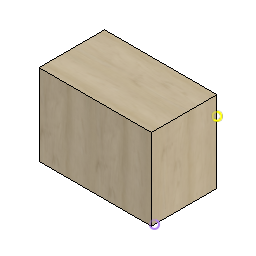
Laminar Casing. v4 (Autodesk Fusion 360 design; units mm, degrees)
Autodesk Fusion 360 part; units mm, degrees
sketch "Sketch1" plane through (0, 0, 0) normal (0, 0, 1) x (1, 0, 0)
  line L0 (25.4, 25.4) -> (939.8, 25.4)
  line L1 (939.8, 25.4) -> (939.8, 533.4)
  line L2 (939.8, 533.4) -> (25.4, 533.4)
  line L3 (25.4, 533.4) -> (25.4, 25.4)
  line L4 (101.6, 381) -> (863.6, 381)
  line L5 (863.6, 381) -> (863.6, 25.4)
  line L6 (863.6, 25.4) -> (101.6, 25.4)
  line L7 (101.6, 25.4) -> (101.6, 381)
  constraint horizontal L0
  constraint vertical L1
  constraint horizontal L2
  constraint vertical L3
  constraint horizontal L4
  constraint vertical L5
  constraint horizontal L6
  constraint vertical L7
  constraint coincident L0 L5.end
extrude "Extrude1" add sketch "Sketch1" against normal blind 508 contours L0 L1 L2 L3 L4 L5 L7
sketch "Sketch2" plane through (0, 0, 0) normal (0, 0, 1) x (1, 0, 0)
  point P0 (939.8, 25.4)
sketch "Sketch3" plane through (0, 0, 0) normal (0, 1, 0) x (1, 0, 0)
  line L0 (939.8, 508) -> (25.4, 508)
  line L1 (25.4, 508) -> (25.4, 0)
  line L2 (25.4, 0) -> (939.8, 0)
  line L3 (939.8, 0) -> (939.8, 508)
  constraint horizontal L0
  constraint vertical L1
  constraint horizontal L2
  constraint vertical L3
extrude "Extrude2" add sketch "Sketch3" along normal blind 25.4
sketch "Sketch4" plane through (0, 0, 0) normal (0, 0, 1) x (1, 0, 0)
box "BoxPrimitive1" add length 533.4 width 914.4 height 152.4 placed x (0, -1, 0) y (1, 0, 0) z (0, 0, 1) at (25.4, 533.4, 0)
sketch "Sketch5" plane through (0, 0, 0) normal (0, 1, 0) x (1, 0, 0)
sketch "Sketch6" plane through (0, 0, 0) normal (0, 0, 1) x (1, 0, 0)
  point P0 (939.8, 533.4)
fillet "Fillet1" radius 24.5618 3 edges at (482.6, 381, -508) (863.6, 203.2, -508) (101.6, 203.2, -508) 1 faces at (609.6, 262.4667, 0)
extrude "Extrude3" add 1 faces at (617.7873, 490.7873, -508) along direction (0, 0, 1) blind 12.7
ref_plane "WorkPlane2" through (482.6, 266.7, -177.8) normal (-1, 0, 0) x (0, 1, 0)
sketch "Sketch7" plane through (0, 533.4, 0) normal (0, 1, 0) x (-1, 0, 0)
  line L0 (-25.4, -508) -> (-25.4, 152.4)
  line L1 (-25.4, 152.4) -> (-939.8, 152.4)
  line L2 (-939.8, 152.4) -> (-939.8, -508)
  line L3 (-939.8, -508) -> (-25.4, -508)
  circle A0 centre (-482.6, -139.7) radius 114.3
  dimension "d14" = 228.6
  measures "d14" diameter of A0
extrude "Extrude4" cut sketch "Sketch7" against normal blind 12.7 contours A0
sketch "Sketch8" plane through (0, 0, 0) normal (0, 0, -1) x (1, 0, 0)
  line L0 (126.1618, -49.9618) -> (126.1618, -356.4382)
  line L1 (126.1618, -356.4382) -> (839.0382, -356.4382)
  line L2 (839.0382, -356.4382) -> (839.0382, -49.9618)
  line L3 (839.0382, -49.9618) -> (126.1618, -49.9618)
  line L4 (622.3, -114.3) -> (342.9, -114.3)
  arc A0 (342.9, -114.3) -> (342.9, -139.7) centre (342.9, -127) ccw
  line L5 (342.9, -139.7) -> (622.3, -139.7)
  arc A1 (622.3, -139.7) -> (622.3, -114.3) centre (622.3, -127) ccw
  line L6 (622.3, -127) -> (342.9, -127) construction
  point P0 (482.6, -127)
  constraint tangent L4 A0
  constraint tangent A0 L5
  constraint parallel L4 L5
  constraint tangent L5 A1
  constraint tangent L4 A1
  constraint parallel L1 L6
  constraint midpoint L6 P0
extrude "Extrude5" cut sketch "Sketch8" against normal blind 12.7 contours L4 A0 L5 A1
sketch "Sketch9" plane through (0, 381, 0) normal (0, -1, 0) x (1, 0, 0)
  line L0 (863.6, -24.5618) -> (101.6, -24.5618)
  line L1 (101.6, -24.5618) -> (101.6, -483.4382)
  line L2 (101.6, -483.4382) -> (863.6, -483.4382)
  line L3 (863.6, -483.4382) -> (863.6, -24.5618)
  line L4 (812.8, -50.8) -> (558.8, -50.8)
  arc A0 (558.8, -50.8) -> (558.8, -101.6) centre (558.8, -76.2) ccw
  line L5 (558.8, -101.6) -> (812.8, -101.6)
  arc A1 (812.8, -101.6) -> (812.8, -50.8) centre (812.8, -76.2) ccw
  line L6 (812.8, -76.2) -> (558.8, -76.2) construction
  line L7 (482.6, -619.76) -> (482.6, 264.16)
  line L8 (406.4, -101.6) -> (152.4, -101.6)
  line L9 (152.4, -50.8) -> (406.4, -50.8)
  arc A2 (152.4, -50.8) -> (152.4, -101.6) centre (152.4, -76.2) ccw
  arc A3 (406.4, -101.6) -> (406.4, -50.8) centre (406.4, -76.2) ccw
  point P0 (685.8, -76.2)
  constraint tangent L4 A0
  constraint tangent A0 L5
  constraint parallel L4 L5
  constraint tangent L5 A1
  constraint tangent L4 A1
  constraint horizontal L6
  constraint midpoint L6 P0
  constraint symmetric L4.start L7 L9.start
  constraint symmetric L4.end L7 L9.end
  constraint symmetric A0.end L7 L8.start
  constraint symmetric L5.end L7 L8.end
  constraint symmetric A0 L7 A3
  constraint symmetric A1 L7 A2
extrude "Extrude6" cut sketch "Sketch9" against normal blind 12.7 contours L4 A0 L5 A1 | L8 L9 A2 A3
shell "Shell1" thickness 12.7 removed faces 0 bodies 1
delete_face "DeleteFace1" 1 faces at (508.2703, 520.7, -194.1581)
delete_face "DeleteFace2" 1 faces at (436.0333, 131.2333, 12.7)
delete_face "DeleteFace3" 1 faces at (728.1333, 393.7, -84.6667)
delete_face "DeleteFace4" 1 faces at (237.0667, 393.7, -67.7333)
